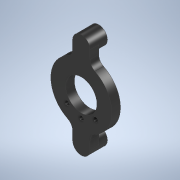
# Autodesk Inventor part: EncoderPinRetainer
Saved by Autodesk Inventor 2020 (Build 240168000, 168)
## iProperties
Created: 2019-06-24
Part Number: EncoderPinRetainer
Material: ABS Plastic
Document SubType Name: Modeling
Designer: Connor
Density: 1.06 g/cm^3
Appearance: Glossy - Black
Author: Connor
Autodesk Inventor part; units mm, degrees
ref_plane "YZ Plane" through (0, 0, 0) normal (1, 0, 0) x (0, 1, 0)
ref_plane "XZ Plane" through (0, 0, 0) normal (0, 1, 0) x (-1, 0, 0)
ref_plane "XY Plane" through (0, 0, 0) normal (0, 0, 1) x (1, 0, 0)
sketch "Sketch1" plane through (0, 0, 0) normal (0, 0, 1) x (1, 0, 0)
  circle A0 centre (0, 0) radius 5.715
  circle A1 centre (0, 0) radius 15.875 construction
  circle A2 centre (0, 15.875) radius 3.175
  circle A3 centre (0, -15.875) radius 3.175
  circle A4 centre (0, 0) radius 11.1125
  line L0 (0, 15.875) -> (0, -15.875) construction
  line L1 (-3.175, 15.875) -> (-3.175, -15.875)
  line L2 (3.175, -15.875) -> (3.175, 15.875)
  arc A5 (3.175, 15.875) -> (-3.175, 15.875) centre (0, 15.875) ccw
  arc A6 (-3.175, -15.875) -> (3.175, -15.875) centre (0, -15.875) ccw
  circle A7 centre (0, -7.366) radius 0.8255
  circle A8 centre (0, 0) radius 7.366 construction
  circle A9 centre (5.2085, -5.2085) radius 0.8255
  circle A10 centre (-5.2085, -5.2085) radius 0.8255
  point P0 (-3.175, 10.6493)
  point P1 (-3.175, -10.6493)
  point P2 (3.175, -10.6493)
  point P3 (3.175, 10.6493)
  point P4 (3.175, 15.875)
  point P5 (3.175, -15.875)
  dimension "d0" = 11.43
  dimension "d1" = 31.75
  dimension "d2" = 6.35
  dimension "d3" = 22.225
  dimension "d6" = 1.651
  dimension "d12" = 14.732
  dimension "d13" = 45
  dimension "d14" = 45
  constraints: 11 centre point, 9 point on circle, 8 end point, 5 tangent, 4 coincident, 3 equal radius, 2 vertical alignment, 1 midpoint, 1 parallel, 1 point on line, 1 vertical
  measures "d0" diameter of A0
  measures "d1" diameter of A1
  measures "d2" diameter of A2
  measures "d3" diameter of A4
  measures "d6" diameter of A7
  measures "d12" diameter of A8
extrude "Extrusion1" add sketch "Sketch1" along normal blind 3.175 contours A0 L2 A4 | A0 L1 A4 L2 | L2 A4 L1 A0 | A0 L1 A4 | A4 L1 A2 L2 | L2 A3 L1 A4 | A2 | A3
extrude "Extrusion2" add sketch "Sketch1" against normal blind 3.175 contours A2 | A3
fillet "Fillet1" radius 3.175 4 edges at (-3.175, -10.6493, 1.5875) (3.175, -10.6493, 1.5875) (-3.175, 10.6493, 1.5875) (3.175, 10.6493, 1.5875)
body "Solid1"
